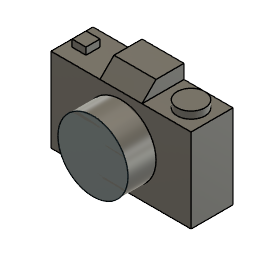
Record 3 (Autodesk Fusion 360 design; units mm, degrees)
part number: 2025-09-27-09-56-54-633
Autodesk Fusion 360 part; units mm, degrees
sketch "Sketch1" plane through (0, 0, 0) normal (0, 0, 1) x (1, 0, 0)
  line L0 (-50, 30) -> (50, 30)
  line L1 (50, 30) -> (50, -30)
  line L2 (50, -30) -> (-50, -30)
  line L3 (-50, -30) -> (-50, 30)
  dimension "d1" = 100
  dimension "d2" = 60
  dimension "d4" = 30
  dimension "d5" = 50
  constraint horizontal L0
  constraint vertical L1
  constraint horizontal L2
  constraint vertical L3
  measures "d1" distance of L0.start L0.end
  measures "d2" distance of L0.start L2.end
  measures "d4" distance of origin L0
  measures "d5" distance of origin L1
extrude "Extrude1" add sketch "Sketch1" along normal blind 30
sketch "Sketch2" plane through (0, 0, 30) normal (0, 0, 1) x (1, 0, 0)
  line L0 (-50, -30) -> (50, -30)
  line L1 (50, -30) -> (50, 30)
  line L2 (50, 30) -> (-50, 30)
  line L3 (-50, 30) -> (-50, -30)
  circle A0 centre (0, 0) radius 25
  dimension "d8" = 50
  constraint coincident A0.centre origin
  measures "d8" diameter of A0
extrude "Extrude2" add sketch "Sketch2" along normal blind 20 contours A0
sketch "Sketch3" plane through (0, 30, 0) normal (0, 1, 0) x (-1, 0, 0)
  line L0 (-50, 0) -> (50, 0)
  line L1 (50, 0) -> (50, 30)
  line L2 (50, 30) -> (-50, 30)
  line L3 (-50, 30) -> (-50, 0)
  line L4 (15, 0) -> (-15, 0)
  line L5 (-15, 0) -> (-15, 30)
  line L6 (-15, 30) -> (15, 30)
  line L7 (15, 30) -> (15, 0)
  constraint horizontal L4
  constraint vertical L5
  constraint horizontal L6
  constraint vertical L7
  constraint coincident L0 L4.start
extrude "Extrude3" add sketch "Sketch3" along normal blind 10 contours L0 L2 L4 L5 L6 L7
sketch "Sketch4" plane through (0, 30, 0) normal (0, 1, 0) x (-1, 0, 0)
  line L0 (-15, 0) -> (-15, 30)
  line L1 (-15, 30) -> (-50, 30)
  line L2 (-50, 30) -> (-50, 0)
  line L3 (-50, 0) -> (-15, 0)
  circle A0 centre (-35, 15) radius 10
  line L4 (45, 10) -> (35, 10)
  line L5 (35, 10) -> (35, 20)
  line L6 (35, 20) -> (45, 20)
  line L7 (45, 20) -> (45, 10)
  line L8 (15, 0) -> (15, 30)
  dimension "d16" = 20
  dimension "d17" = 20
  dimension "d18" = 20
  constraint horizontal L4
  constraint vertical L5
  constraint horizontal L6
  constraint vertical L7
  measures "d16" diameter of A0
  measures "d17" distance of L0 A0.centre
  measures "d18" distance of L5 L8
extrude "Extrude4" add sketch "Sketch4" along normal blind 5 contours A0 | L4 L5 L6 L7
sketch "Sketch5" plane through (15, 0, 0) normal (1, 0, 0) x (0, 0, -1)
  line L0 (-30, 30) -> (0, 30)
  line L1 (0, 30) -> (0, 40)
  line L2 (0, 40) -> (-30, 40)
  line L3 (-30, 40) -> (-30, 30)
  line L4 (-30, 40) -> (-30, 30)
  line L5 (-30, 30) -> (-20, 40)
  line L6 (-20, 40) -> (-30, 40)
  constraint coincident L2.end L3.start
  constraint coincident L0.start L3.end
  constraint coincident L2 L5.end
extrude "Extrude5" cut sketch "Sketch5" against normal blind 35 contours L2 L3 L4 L5 L6
sketch "Sketch6" plane through (0, 0, 50) normal (0, 0, 1) x (1, 0, 0)
  circle A0 centre (0, 0) radius 25
